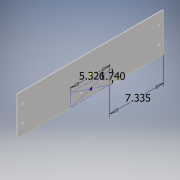
# Autodesk Inventor part: nmt_sidepanel_20in
Saved by Autodesk Inventor 2017 (Build 210142000, 142)
## iProperties
Created: 2017-02-19
Part Number: nmt_sidepanel_20in
Material: Generic
Document SubType Name: Modeling
Designer: Zara
Density: 1 g/cm^3
Appearance: Default
Author: Zara
Autodesk Inventor part; units mm, degrees
ref_plane "YZ Plane" through (0, 0, 0) normal (1, 0, 0) x (0, 1, 0)
ref_plane "XZ Plane" through (0, 0, 0) normal (0, 1, 0) x (-1, 0, 0)
ref_plane "XY Plane" through (0, 0, 0) normal (0, 0, 1) x (1, 0, 0)
sketch "Sketch1" plane through (0, 0, 0) normal (1, 0, 0) x (0, 1, 0)
  line L0 (-66.294, 254) -> (66.294, 254)
  line L1 (66.294, 254) -> (66.294, -254)
  line L2 (66.294, -254) -> (-66.294, -254)
  line L3 (-66.294, -254) -> (-66.294, 254)
  line L4 (-66.294, 254) -> (66.294, -254) construction
  line L5 (66.294, 254) -> (-66.294, -254) construction
  point P0 (0, 0)
  dimension "d0" = 508
  dimension "d1" = 132.588
  constraints: 12 end point, 2 midpoint, 2 parallel, 1 horizontal, 1 perpendicular
  measures "d0" distance of L0.end L1.end
  measures "d1" distance of L1.end L2.end
extrude "Extrusion1" add sketch "Sketch1" along normal blind 3.175
sketch "Sketch2" plane through (3.175, 0, 0) normal (1, 0, 0) x (0, 0, -1)
  line L0 (-67.5894, -66.294) -> (67.691, -66.294) construction
  line L1 (67.691, -66.294) -> (67.691, -22.098) construction
  line L2 (67.691, -22.098) -> (-67.5894, -22.098) construction
  line L3 (-67.5894, -22.098) -> (-67.5894, -66.294) construction
  line L4 (-67.5894, -66.294) -> (67.691, -22.098) construction
  line L5 (67.691, -66.294) -> (-67.5894, -22.098) construction
  line L6 (254, -66.294) -> (254, 66.294) construction
  line L7 (-254, -66.294) -> (254, -66.294) construction
  point P0 (0, 0)
  point P1 (0.0508, -44.196)
  point P2 (10.6003, -66.294)
  dimension "d4" = 135.2804
  dimension "d5" = 44.196
  dimension "d6" = 186.309
  constraints: 12 end point, 2 midpoint, 2 parallel, 2 point on line, 1 horizontal, 1 perpendicular
  measures "d4" distance of L1.end L2.end
  measures "d5" distance of L0.end L1.end
  measures "d6" distance between parallel lines of L6 L1
sketch "Sketch3" plane through (3.175, 0, 0) normal (1, 0, 0) x (0, 0, -1)
  line L0 (-33.7566, -40.005) -> (33.8582, -40.005) construction
  line L1 (-254, -66.294) -> (254, -66.294) construction
  line L2 (67.691, -66.294) -> (67.691, -22.098) construction
  line L3 (-67.5894, -22.098) -> (-67.5894, -66.294) construction
  point P0 (0, 0)
  dimension "d7" = 26.289
  dimension "d17" = 33.8328
  dimension "d18" = 33.8328
  constraints: 2 end point, 1 horizontal
  measures "d7" distance between parallel lines of L0 L1
  measures "d17" distance from line of L2 L0.end
  measures "d18" distance from line of L3 L0.start
hole "Hole1" at (3.175, -40.005, 33.7566) at (3.175, -40.005, -33.8582) direction (-1, 0, 0) diameter 4.4958 end through all clearance for "Countersunk Flat Head Screw ISO 2009/7046" size "M4" standard "ISO"
sketch "brackets" plane through (3.175, 0, 0) normal (1, 0, 0) x (0, 0, -1)
  line L0 (254, -66.294) -> (254, 66.294) construction
  line L1 (249.428, 54.61) -> (230.378, 54.61) construction
  line L2 (230.378, 54.61) -> (230.378, -54.61) construction
  line L3 (230.378, -54.61) -> (249.428, -54.61) construction
  line L4 (249.428, -54.61) -> (249.428, 54.61) construction
  line L5 (254, 66.294) -> (-254, 66.294) construction
  line L6 (-254, 66.294) -> (-254, -66.294) construction
  line L7 (-249.428, 54.61) -> (-230.378, 54.61) construction
  line L8 (-230.378, 54.61) -> (-230.378, -54.61) construction
  line L9 (-230.378, -54.61) -> (-249.428, -54.61) construction
  line L10 (-249.428, -54.61) -> (-249.428, 54.61) construction
  point P0 (0, 0)
  point P1 (-236.3724, 29.21)
  point P2 (-236.3724, -29.21)
  point P3 (236.3724, 29.21)
  point P4 (236.3724, -29.21)
  dimension "d20" = 19.05
  dimension "d21" = 109.22
  dimension "d22" = 11.684
  dimension "d23" = 19.05
  dimension "d24" = 109.22
  dimension "d25" = 11.684
  dimension "d26" = 25.4
  dimension "d27" = 5.9944
  dimension "d28" = 25.4
  dimension "d29" = 5.9944
  dimension "d30" = 25.4
  dimension "d31" = 5.9944
  dimension "d32" = 25.4
  dimension "d33" = 5.9944
  dimension "d41" = 4.572
  dimension "d42" = 4.572
  constraints: 16 end point, 4 parallel, 2 horizontal, 2 perpendicular
  measures "d20" distance of L1.start L1.end
  measures "d21" distance of L1.end L2.end
  measures "d22" distance between parallel lines of L5 L1
  measures "d23" distance of L7.start L7.end
  measures "d24" distance of L7.end L8.end
  measures "d25" distance between parallel lines of L5 L7
  measures "d26" distance from line of point (-236.372, 29.21) L7
  measures "d27" distance from line of L8 point (-236.372, 29.21)
  measures "d28" distance from line of L9 point (-236.372, -29.21)
  measures "d29" distance from line of L8 point (-236.372, -29.21)
  measures "d30" distance from line of point (236.372, 29.21) L1
  measures "d31" distance from line of L2 point (236.372, 29.21)
  measures "d32" distance from line of L3 point (236.372, -29.21)
  measures "d33" distance from line of L2 point (236.372, -29.21)
  measures "d41" distance between parallel lines of L6 L10
  measures "d42" distance between parallel lines of L0 L4
hole "Hole2" at (3.175, 29.21, 236.3724) at (3.175, -29.21, 236.3724) at (3.175, 29.21, -236.3724) at (3.175, -29.21, -236.3724) direction (-1, 0, 0) diameter 4.2926 end through all countersink diameter 9.398 countersink angle 90 clearance for "Countersunk Flat Head Screw ISO 2009/7046" size "M4" standard "ISO"
body "Solid1"
